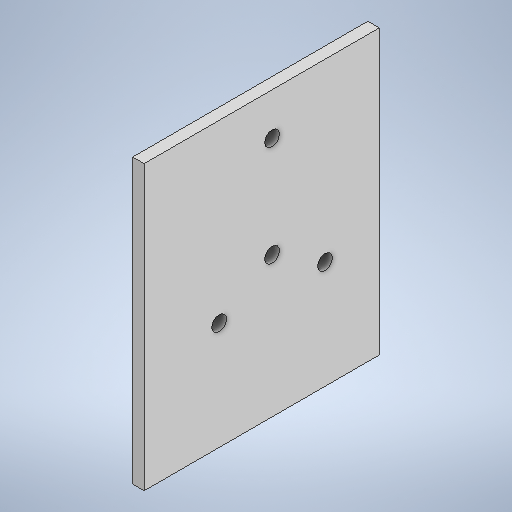
# Autodesk Inventor part: bigwall
Saved by Autodesk Inventor 2025.1 (Build 291241000, 241)
## iProperties
Created: 2025-11-11
Part Number: bigwall
Material: Generic
Document SubType Name: Modeling
Designer: mukund
Density: 1 g/cm^3
Appearance: Default
Author: mukund
Autodesk Inventor part; units mm, degrees
ref_plane "YZ Plane" through (0, 0, 0) normal (1, 0, 0) x (0, 1, 0)
ref_plane "XZ Plane" through (0, 0, 0) normal (0, 1, 0) x (-1, 0, 0)
ref_plane "XY Plane" through (0, 0, 0) normal (0, 0, 1) x (1, 0, 0)
sketch "Sketch1" plane through (0, 0, 0) normal (1, 0, 0) x (0, 1, 0)
  line L0 (0, 0) -> (247, 0)
  line L1 (247, 0) -> (247, -205)
  line L2 (247, -205) -> (0, -205)
  line L3 (0, -205) -> (0, 0)
  circle A0 centre (93.85, -65.35) radius 6.4
  circle A1 centre (93.85, -157.65) radius 6.4
  line L4 (93.85, -65.35) -> (93.85, -157.65)
  circle A2 centre (122.4, -111.5) radius 6.4
  line L5 (122.4, -111.5) -> (116, -111.5)
  line L6 (116, -111.5) -> (210.35, -111.5)
  circle A3 centre (210.35, -111.5) radius 6.4
  point P0 (122.35, 111.5)
  dimension "d5" = 12.8
  dimension "d0" = 247
  dimension "d1" = 205
  dimension "d3" = 12.8
  dimension "d4" = 92.3
  dimension "d6" = 94.35
  dimension "d7" = 12.8
  dimension "d10" = 12.8
  constraints: 14 end point, 5 coincident, 3 centre point, 2 horizontal, 2 parallel, 1 horizontal alignment, 1 perpendicular, 1 point on line, 1 vertical, 2 other
  measures "d0" distance of L1.end L2.end
  measures "d1" distance of L0.end L1.end
  measures "d3" diameter of A1
  measures "d4" distance of L4.start L4.end
  measures "d6" distance of L5.end L6.end
  measures "d7" diameter of A3
  measures "d10" diameter of A0
extrude "Extrusion1" add sketch "Sketch1" along normal blind 10
body "Solid1"
